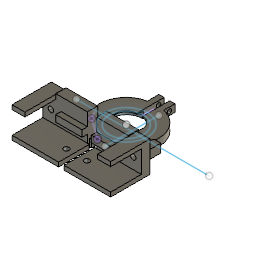
Tuisnlang to body koppelstuk (Autodesk Fusion 360 design; units mm, degrees)
part number: 2025-12-09-10-40-52-901
Autodesk Fusion 360 part; units mm, degrees
sketch "Sketch1" plane through (0, 0, 0) normal (0, 0, 1) x (1, 0, 0)
  circle A0 centre (0, 0) radius 25
  dimension "d1" = 50
  constraint coincident A0.centre origin
  measures "d1" diameter of A0
extrude "Extrude1" add sketch "Sketch1" along normal blind 2.6 makes body 1
sketch "Sketch2" plane through (0, 0, 2.6) normal (0, 0, 1) x (-1, 0, 0)
  circle A0 centre (0, 0) radius 25
  circle A1 centre (0, 0) radius 15
  dimension "d4" = 30
  constraint coincident A0.centre A1.centre
  measures "d4" diameter of A1
extrude "Extrude2" cut sketch "Sketch2" against normal blind 2.6 contours A1 bodies 1
sketch "Sketch3" plane through (0, 0, 0) normal (0, 1, 0) x (1, 0, 0)
sketch "Sketch5" plane through (0, 0, 0) normal (0, 0, 1) x (1, 0, 0)
  line L0 (-21.0001, -11.0728) -> (-21.84, -24.9305)
  line L1 (-21.84, -24.9305) -> (-16.242, -33.6943)
  line L2 (-16.242, -33.6943) -> (-1.8162, -24.4796)
  line L3 (-21.0001, -11.0728) -> (-1.8162, -24.4796)
  line L4 (-1.8162, -24.4796) -> (-1.8162, -34)
  line L5 (-1.8162, -34) -> (-31, -34)
  line L6 (-31, -34) -> (-31, -4.0843)
  line L7 (-31, -4.0843) -> (-25, -4.0843)
  line L8 (-25, -4.0843) -> (-21.0001, -11.0728)
  constraint perpendicular L1 L2
  constraint vertical L4
  constraint perpendicular L4 L5
  constraint perpendicular L5 L6
  constraint perpendicular L6 L7
extrude "Extrude3" add sketch "Sketch5" along normal blind 8 bodies 1
sketch "Sketch6" plane through (0, 0, 2.6) normal (0, 0, 1) x (-1, 0, 0)
  arc A0 (1.8162, 24.9339) -> (24.5053, 4.9486) centre (0, 0) ccw
  circle A1 centre (0, 0) radius 15
  circle A2 centre (32.676, 4.348) radius 1
  line L0 (24.5053, 4.9486) -> (21.0001, 11.0728)
  line L1 (21.0001, 11.0728) -> (1.8162, 24.4796)
  line L2 (1.8162, 24.4796) -> (1.8162, 24.9339)
  dimension "d9" = 2
  measures "d9" diameter of A2
extrude "Extrude4" cut sketch "Sketch6" against normal blind 2.6 contours A2 bodies 1
sketch "Sketch8" plane through (0, 0, 0) normal (0, 0, 1) x (1, 0, 0)
  line L0 (0, 25) -> (0, -25.7353)
  line L1 (0, -25.7353) -> (12.6085, -23.4951)
  line L2 (12.6085, -23.4951) -> (25, -10.7696)
  line L3 (25, -10.7696) -> (25, 9.1686)
  line L4 (25, 9.1686) -> (14.4225, 21.7368)
  line L5 (14.4225, 21.7368) -> (4.3268, 26.0635)
  line L6 (4.3268, 26.0635) -> (0, 25)
  constraint vertical L0
  constraint parallel L0 L3
extrude "Extrude5" cut sketch "Sketch8" along normal blind 19 bodies 1
sketch "Sketch9" plane through (0, 0, 0) normal (0, 0, 1) x (1, 0, 0)
  line L0 (4.9276, 25.1738) -> (4.9276, -24.4237)
  line L1 (-46, 0) -> (76.5197, 0)
  constraint vertical L0
  constraint horizontal L1
sketch "Sketch10" plane through (0, 0, 0) normal (0, 0, 1) x (1, 0, 0)
  spline S0 degree 5 poles (-0.4071, 24.1491) (-0.4918, 24.0205) (-0.6962, 23.8243) (-1.102, 23.7009) (-1.822, 23.7859) (-2.9658, 23.9832) (-4.2807, 23.9855) (-5.6641, 23.6781) (-7.0121, 23.0757) (-8.2499, 22.2797) (-9.3589, 21.4375) (-10.4145, 20.6984) (-11.5168, 20.2085) (-12.7525, 20.094) (-14.1577, 20.4469) (-15.6684, 21.3064) (-17.1289, 22.6564) (-18.3401, 24.4341) (-19.0952, 26.5352) (-19.2214, 28.8193) (-18.6168, 31.1155) (-17.296, 33.2264) (-15.3689, 34.9492) (-13.0093, 36.0992) (-10.4289, 36.5324) (-7.8486, 36.1699) (-5.4721, 35.0198) (-3.4561, 33.2063) (-1.8896, 30.981) (-0.8095, 28.6573) (-0.2122, 26.5558) (-0.0948, 25.268) (-0.1875, 24.5959) (-0.3223, 24.2778) (-0.4071, 24.1491) knots 0 0 0 0 0 0 0.033333 0.066667 0.1 0.133333 0.166667 0.2 0.233333 0.266667 0.3 0.333333 0.366667 0.4 0.433333 0.466667 0.5 0.533333 0.566667 0.6 0.633333 0.666667 0.7 0.733333 0.766667 0.8 0.833333 0.866667 0.9 0.933333 0.966667 1 1 1 1 1 1
  line L0 (-5.9786, 23.8802) -> (-11.3635, 20.0197)
  line L1 (-46, 0) -> (76.5197, 0)
  spline S1 degree 5 poles (-0.4071, -24.1491) (-0.4918, -24.0205) (-0.6962, -23.8243) (-1.102, -23.7009) (-1.822, -23.7859) (-2.9658, -23.9832) (-4.2807, -23.9855) (-5.6641, -23.6781) (-7.0121, -23.0757) (-8.2499, -22.2797) (-9.3589, -21.4375) (-10.4145, -20.6984) (-11.5168, -20.2085) (-12.7525, -20.094) (-14.1577, -20.4469) (-15.6684, -21.3064) (-17.1289, -22.6564) (-18.3401, -24.4341) (-19.0952, -26.5352) (-19.2214, -28.8193) (-18.6168, -31.1155) (-17.296, -33.2264) (-15.3689, -34.9492) (-13.0093, -36.0992) (-10.4289, -36.5324) (-7.8486, -36.1699) (-5.4721, -35.0198) (-3.4561, -33.2063) (-1.8896, -30.981) (-0.8095, -28.6573) (-0.2122, -26.5558) (-0.0948, -25.268) (-0.1875, -24.5959) (-0.3223, -24.2778) (-0.4071, -24.1491) knots 0 0 0 0 0 0 0.033333 0.066667 0.1 0.133333 0.166667 0.2 0.233333 0.266667 0.3 0.333333 0.366667 0.4 0.433333 0.466667 0.5 0.533333 0.566667 0.6 0.633333 0.666667 0.7 0.733333 0.766667 0.8 0.833333 0.866667 0.9 0.933333 0.966667 1 1 1 1 1 1
  line L2 (0.3754, 25.3361) -> (-1.1896, 22.9622)
  line L3 (0.3754, -25.3361) -> (-1.1896, -22.9622)
  line L4 (-5.9786, -23.8802) -> (-11.3635, -20.0197)
  point P0 (-3.0127, 23.9362)
  point P1 (-8.6711, 21.9499)
  point P2 (-13.3389, 20.2988)
  point P3 (-19, 29.1318)
  point P4 (-6, 35.1318)
  point P5 (-3.0127, -23.9362)
  point P6 (-8.6711, -21.9499)
  point P7 (-13.3389, -20.2988)
  point P8 (-19, -29.1318)
  point P9 (-6, -35.1318)
  constraint midpoint P1 L0
  constraint midpoint S0.start L2
  constraint symmetric S0.start L1 S1.start
  constraint symmetric P0 L1 P5
  constraint symmetric P1 L1 P6
  constraint symmetric P2 L1 P7
  constraint symmetric P3 L1 P8
  constraint symmetric P4 L1 P9
  constraint symmetric L0.start L1 L4.start
  constraint symmetric L0.end L1 L4.end
  constraint symmetric L1 L2.start L3.start
  constraint symmetric L1 L2.end L3.end
sketch "Sketch13" plane through (0, 0, 0) normal (0, 0, 1) x (1, 0, 0)
  line L0 (9.9066, 24.8111) -> (24.4111, 20.3394)
  line L1 (24.4111, 20.3394) -> (30.2441, 35.4836)
  line L2 (30.2441, 35.4836) -> (10.9741, 35.4836)
  line L3 (10.9741, 35.4836) -> (9.9066, 24.8111)
  line L4 (-46, 0) -> (76.5197, 0)
  line L5 (30.2441, -35.4836) -> (10.9741, -35.4836)
  line L6 (10.9741, -35.4836) -> (9.9066, -24.8111)
  line L7 (9.9066, -24.8111) -> (24.4111, -20.3394)
  line L8 (24.4111, -20.3394) -> (30.2441, -35.4836)
  constraint horizontal L2
  constraint symmetric L0.start L4 L6.end
  constraint symmetric L0.end L4 L7.end
  constraint symmetric L1.end L4 L5.start
  constraint symmetric L2.end L4 L5.end
sketch "Sketch19" plane through (0, 0, 2.6) normal (0, 0, 1) x (-1, 0, 0)
  line L0 (0, 25) -> (0, 15)
  arc A0 (0, -15) -> (0, 15) centre (0, 0) ccw
  arc A1 (0, -25) -> (24.5053, 4.9486) centre (0, 0) ccw
  circle A2 centre (0, 0) radius 15.7
  line L1 (0, -15) -> (0, -25)
  line L2 (24.5053, 4.9486) -> (21.0001, 11.0728)
  line L3 (21.0001, 11.0728) -> (1.8162, 24.4796)
  line L4 (1.8162, 24.4796) -> (1.8162, 24.9339)
  arc A3 (1.8162, 24.9339) -> (0, 25) centre (0, 0) ccw
  dimension "d25" = 31.4
  measures "d25" diameter of A2
sketch "Sketch20" plane through (0, 0, 2.6) normal (0, 0, 1) x (-1, 0, 0)
  line L0 (0, 25) -> (0, 15)
  arc A0 (0, -15) -> (0, 15) centre (0, 0) ccw
  arc A1 (0, -25) -> (24.5053, 4.9486) centre (0, 0) ccw
  circle A2 centre (0, 0) radius 19.4774
  circle A3 centre (0, 0) radius 15.7
  line L1 (0, -15) -> (0, -25)
  line L2 (24.5053, 4.9486) -> (21.0001, 11.0728)
  line L3 (21.0001, 11.0728) -> (1.8162, 24.4796)
  line L4 (1.8162, 24.4796) -> (1.8162, 24.9339)
  arc A4 (1.8162, 24.9339) -> (0, 25) centre (0, 0) ccw
  dimension "d30" = 31.4
  measures "d30" diameter of A3
extrude "Extrude12" add sketch "Sketch20" along normal blind 3.3 contours L0 A2 A3 L1 picked at (1.6688, 18.0989) bodies 1
sketch "Sketch21" plane through (0, 0, 5.9) normal (0, 0, 1) x (-1, 0, 0)
  arc A0 (0, -19.4774) -> (0, 19.4774) centre (0, 0) ccw
  line L0 (0, 19.4774) -> (0, 15.7)
  arc A1 (0, -15.7) -> (0, 15.7) centre (0, 0) ccw
  line L1 (0, -15.7) -> (0, -19.4774)
  circle A2 centre (0, 0) radius 19.4774
  constraint concentric A0 A2
extrude "Extrude13" add sketch "Sketch21" along normal blind 1 bodies 1
sketch "Sketch22" plane through (0, 0, 6.9) normal (0, 0, 1) x (-1, 0, 0)
  circle A0 centre (0, 0) radius 19.4774
  circle A1 centre (0, 0) radius 9.85
  dimension "d35" = 19.7
  constraint coincident A0.centre A1.centre
  measures "d35" diameter of A1
extrude "Extrude14" cut sketch "Sketch22" against normal blind 2 contours A1 bodies 1
extrude "Extrude15" add sketch "Sketch20" along normal blind 4.3 contours L0 A1 A2 L1 L2 L3 L4 A4 bodies 1
sketch "Sketch24" plane through (0, 0, 6.9) normal (0, 0, 1) x (-1, 0, 0)
  circle A0 centre (0, 0) radius 9.85
  arc A1 (0, 19.4774) -> (0, -19.4774) centre (0, 0) ccw
  line L0 (0, 24) -> (6, 24)
  line L1 (6, 24) -> (6, 32)
  line L2 (6, 32) -> (0, 32)
  line L3 (0, 32) -> (0, 24)
  line L4 (0, -19.4774) -> (0, -25)
  arc A2 (0, -25) -> (24.5053, 4.9486) centre (0, 0) ccw
  line L5 (0, 25) -> (0, 19.4774)
  line L6 (24.5053, 4.9486) -> (21.0001, 11.0728)
  line L7 (21.0001, 11.0728) -> (1.8162, 24.4796)
  line L8 (1.8162, 24.4796) -> (1.8162, 24.9339)
  arc A3 (1.8162, 24.9339) -> (0, 25) centre (0, 0) ccw
  constraint horizontal L0
  constraint vertical L1
  constraint horizontal L2
  constraint vertical L3
extrude "Extrude16" add sketch "Sketch24" against normal blind 6.9 contours L0 L3 L5 L7 L8 A3 | L0 L1 L2 L3 L7 L8 A3 bodies 1
sketch "Sketch25" plane through (0, 0, 0) normal (0, 0, 1) x (1, 0, 0)
  line L0 (0, 24.3391) -> (-5, 24.3391)
  line L1 (-5, 24.3391) -> (-5, 35.1439)
  line L2 (-5, 35.1439) -> (0, 35.1439)
  line L3 (0, 35.1439) -> (0, 24.3391)
  constraint horizontal L0
  constraint vertical L1
  constraint horizontal L2
  constraint vertical L3
extrude "Extrude17" add sketch "Sketch25" along normal blind 6.9 bodies 1
sketch "Sketch28" plane through (-31, 0, 0) normal (-1, 0, 0) x (0, -1, 0)
  line L0 (4.0843, 0) -> (34, 0)
  line L1 (34, 0) -> (34, 8)
  line L2 (34, 8) -> (4.0843, 8)
  line L3 (4.0843, 8) -> (4.0843, 0)
  line L4 (34, 8) -> (31, 8)
  line L5 (31, 8) -> (31, 0)
  line L6 (31, 0) -> (34, 0)
  line L7 (34, 0) -> (34, 8)
  constraint horizontal L4
  constraint vertical L5
  constraint horizontal L6
  constraint vertical L7
  constraint coincident L0 L5.end
  constraint coincident L1.end L2.start
extrude "Extrude19" add sketch "Sketch28" along normal blind 9 contours L0 L1 L2 L4 L5 L6 L7 bodies 1
sketch "Sketch29" plane through (0, -34, 0) normal (0, -1, 0) x (1, 0, 0)
  line L0 (-1.8162, 8) -> (-40, 8)
  line L1 (-40, 8) -> (-40, 0)
  line L2 (-40, 0) -> (-1.8162, 0)
  line L3 (-1.8162, 0) -> (-1.8162, 8)
  line L4 (-40, 4) -> (-31, 4)
  line L5 (-31, 4) -> (-31, 0)
  line L6 (-31, 0) -> (-40, 0)
  line L7 (-40, 0) -> (-40, 4)
  constraint horizontal L4
  constraint vertical L5
  constraint horizontal L6
  constraint vertical L7
  constraint coincident L2 L5.end
  constraint midpoint L1 L4.start
extrude "Extrude20" add sketch "Sketch29" along normal blind 12 contours L1 L2 L4 L5 L6 L7 bodies 1
sketch "Sketch30" plane through (0, 0, 8) normal (0, 0, 1) x (-1, 0, 0)
  line L0 (25, 4.0843) -> (31, 4.0843)
  line L1 (31, 4.0843) -> (31, 31)
  line L2 (31, 31) -> (40, 31)
  line L3 (40, 31) -> (40, 34)
  line L4 (40, 34) -> (1.8162, 34)
  line L5 (1.8162, 34) -> (1.8162, 24.4796)
  line L6 (1.8162, 24.4796) -> (21.0001, 11.0728)
  line L7 (21.0001, 11.0728) -> (25, 4.0843)
  line L8 (31, 31) -> (40, 31)
  line L9 (40, 31) -> (40, 34)
  line L10 (40, 34) -> (31, 34)
  line L11 (31, 34) -> (31, 31)
  constraint horizontal L8
  constraint vertical L9
  constraint horizontal L10
  constraint vertical L11
  constraint coincident L3.end L4.start
  constraint coincident L1.end L2.start
extrude "Extrude21" add sketch "Sketch30" along normal blind 16.4 contours L2 L3 L4 L8 L9 L10 L11 bodies 1
sketch "Sketch31" plane through (0, 0, 24.4) normal (0, 0, 1) x (-1, 0, 0)
  line L0 (31, 34) -> (31, 31)
  line L1 (31, 31) -> (40, 31)
  line L2 (40, 31) -> (40, 34)
  line L3 (40, 34) -> (31, 34)
  line L4 (31, 31) -> (40, 31)
  line L5 (40, 31) -> (40, 34)
  line L6 (40, 34) -> (31, 34)
  line L7 (31, 34) -> (31, 31)
  constraint horizontal L4
  constraint vertical L5
  constraint horizontal L6
  constraint vertical L7
  constraint coincident L2.end L3.start
  constraint coincident L0.end L1.start
extrude "Extrude22" add sketch "Sketch31" along normal blind 4 bodies 1
sketch "Sketch32" plane through (0, -34, 0) normal (0, -1, 0) x (1, 0, 0)
  line L0 (-40, 4) -> (-31, 4)
  line L1 (-1.8162, 0) -> (-1.8162, 8)
  line L2 (-1.8162, 8) -> (-31, 8)
  line L3 (-31, 8) -> (-31, 28.4)
  line L4 (-31, 28.4) -> (-40, 28.4)
  line L5 (-40, 28.4) -> (-40, 4)
  line L6 (-40, 28.4) -> (-31, 28.4)
  line L7 (-31, 28.4) -> (-31, 24.4)
  line L8 (-31, 24.4) -> (-40, 24.4)
  line L9 (-40, 24.4) -> (-40, 28.4)
  line L10 (-31, 4) -> (-31, 0)
  line L11 (-31, 0) -> (-1.8162, 0)
  dimension "d54" = 4
  constraint horizontal L6
  constraint vertical L7
  constraint horizontal L8
  constraint vertical L9
  constraint coincident L4.end L5.start
  measures "d54" distance of L4.end L8.end
extrude "Extrude23" add sketch "Sketch32" along normal blind 12 contours L3 L4 L5 L6 L7 L8 L9 bodies 1
sketch "Sketch34" plane through (0, 0, 6.9) normal (0, 0, 1) x (-1, 0, 0)
  arc A0 (5, -24.4949) -> (24.5053, 4.9486) centre (0, 0) ccw
  line L0 (24.5053, 4.9486) -> (21.0001, 11.0728)
  line L1 (21.0001, 11.0728) -> (1.8162, 24.4796)
  line L2 (1.8162, 24.4796) -> (1.8162, 32)
  line L3 (1.8162, 32) -> (0, 32)
  line L4 (0, 32) -> (0, 19.4774)
  arc A1 (0, 19.4774) -> (0, -19.4774) centre (0, 0) ccw
  line L5 (0, -19.4774) -> (0, -35.1439)
  line L6 (0, -35.1439) -> (5, -35.1439)
  line L7 (5, -35.1439) -> (5, -24.4949)
  circle A2 centre (0, 0) radius 9.85
  line L8 (0, 25) -> (-19.4774, 25)
  line L9 (-19.4774, 25) -> (-19.4774, -22.8796)
  line L10 (-19.4774, -22.8796) -> (0, -22.8796)
  line L11 (0, -22.8796) -> (0, 25)
  constraint horizontal L8
  constraint vertical L9
  constraint horizontal L10
  constraint vertical L11
  constraint coincident L4 L8.start
extrude "Extrude24" cut sketch "Sketch34" against normal blind 3 contours A1 L5 L9 L10 L11 | A1 A2 L11 | L4 A1 L8 L9 L11 | A2 L11 picked at (-2.567, 2.0471) bodies 1
sketch "Sketch35" plane through (0, 0, 8) normal (0, 0, 1) x (-1, 0, 0)
  line L0 (31, 31) -> (31, 34)
  line L1 (31, 34) -> (1.8162, 34)
  line L2 (1.8162, 34) -> (1.8162, 24.4796)
  line L3 (1.8162, 24.4796) -> (21.0001, 11.0728)
  line L4 (21.0001, 11.0728) -> (25, 4.0843)
  line L5 (25, 4.0843) -> (31, 4.0843)
  line L6 (31, 4.0843) -> (31, 31)
  line L7 (1.8162, 24.4796) -> (31, 24.4796)
  line L8 (31, 24.4796) -> (31, 34)
  line L9 (31, 34) -> (1.8162, 34)
  line L10 (1.8162, 34) -> (1.8162, 24.4796)
  constraint horizontal L7
  constraint vertical L8
  constraint horizontal L9
  constraint vertical L10
  constraint coincident L0.end L1.start
  constraint coincident L2.end L3.start
extrude "Extrude25" add sketch "Sketch35" along normal blind 21 contours L0 L1 L2 L6 L7 L8 L9 L10 bodies 1
sketch "Sketch36" plane through (0, -34, 0) normal (0, -1, 0) x (1, 0, 0)
  line L0 (-31, 24.4) -> (-40, 24.4)
  line L1 (-40, 24.4) -> (-40, 4)
  line L2 (-40, 4) -> (-31, 4)
  line L3 (-31, 4) -> (-31, 0)
  line L4 (-31, 0) -> (-1.8162, 0)
  line L5 (-1.8162, 0) -> (-1.8162, 29)
  line L6 (-1.8162, 29) -> (-31, 29)
  line L7 (-31, 29) -> (-31, 28.4)
  line L8 (-31, 28.4) -> (-31, 24.4)
  line L9 (-40, 14.2) -> (-1.8162, 14.2)
  line L10 (-26.0013, 17.2) -> (-26.0013, 10.4445)
  line L11 (-26.0013, 17.2) -> (-1.8162, 17.2)
  line L12 (-1.8162, 17.2) -> (-1.8162, 11.2)
  line L13 (-1.8162, 11.2) -> (-26.0013, 11.2)
  line L14 (-26.0013, 11.2) -> (-26.0013, 10.4445)
  line L15 (-1.8162, 10.4445) -> (-1.8162, 11.2)
  line L16 (-31, 24.4) -> (-1.8162, 24.4)
  line L17 (-1.8162, 24.4) -> (-1.8162, 17.2)
  line L18 (-31, 4) -> (-1.8162, 4)
  line L19 (-1.8162, 4) -> (-1.8162, 11.2)
  dimension "d61" = 6
  dimension "d62" = 7.2
  constraint midpoint L1 L9.start
  constraint coincident L5 L9.end
  constraint perpendicular L5 L9
  constraint perpendicular L9 L10
  constraint coincident L5 L11.end
  constraint perpendicular L5 L11
  constraint perpendicular L9 L12
  constraint horizontal L13
  constraint coincident L0.start L8.end
  constraint coincident L5 L16.end
  constraint perpendicular L5 L16
  constraint coincident L2.end L3.start
  constraint coincident L5 L18.end
  constraint perpendicular L5 L18
  measures "d61" distance of L11.end L12.end
  measures "d62" distance of L11.end L16.end
extrude "Extrude26" add sketch "Sketch36" along normal blind 5 contours L5 L9 L10 L11 L12 | L5 L9 L10 L12 L13 bodies 1
mirror "Mirror2" about plane through (0, 0, 0) normal (1, 0, 0) of bodies 1 makes body 2
move_body "Move3" bodies 2 to x (1, 0, 0) y (0, 1, 0) z (0, 0, 1) at (5, 0, 0)
hole "Hole1" at (10, 29.8194, 3.45) direction (-1, 0, 0) diameter 4 depth 20 tip angle 118 bodies 1 2
hole "Hole2" at (-35.5, -31, 14.2) direction (0, -1, 0) diameter 5 depth 6 tip angle 118 bodies 1
hole "Hole3" at (40.472, -31, 14.2) direction (0, -1, 0) diameter 5 depth 5 tip angle 118 bodies 2
extrude "Extrude27" add 2 faces at (-35.5, -31, 24.5) (40.4907, -31, 3.9) along direction (0, 1, 0) blind 5 on bodies 1 2 bodies 1 2
extrude "Extrude28" add 1 faces at (-40, -28.6667, 10.8) along direction (-1, 0, 0) blind 3 on bodies 1 bodies 1
extrude "Extrude29" add 1 faces at (45, -28.6667, 10.8) along direction (1, 0, 0) blind 3 on bodies 2 bodies 2
extrude "Extrude30" add 4 faces at (44, -46, 1.3333) (40, -46, 27.0667) (-35, -46, 27.0667) (-35, -46, 2.6667) along direction (0, -1, 0) blind 16.4 on bodies 1 2 bodies 2 1
extrude "Extrude31" add 1 faces at (-31, -43.4667, 2.6667) along direction (1, 0, 0) blind 31 on bodies 1 bodies 1
extrude "Extrude32" add 1 faces at (36, -43.4667, 2.6667) along direction (-1, 0, 0) blind 31 on bodies 2 bodies 2
hole "Hole6" at (42, -40.255, 0) direction (0, 0, 1) diameter 5 depth 6 tip angle 118 bodies 2
hole "Hole7" at (-37, -40.2, 0) direction (0, 0, 1) diameter 5 depth 6 tip angle 118 bodies 1
move_face "MoveFace1" to x (1, 0, 0) y (0, 1, 0) z (0, 0, 1) at (-30, -8, 0) 1 faces at (42.2489, -37.7674, 2.6667) on bodies 2
move_face "MoveFace2" to x (1, 0, 0) y (0, 1, 0) z (0, 0, 1) at (30, -8, 0) 1 faces at (-36.7511, -37.7124, 2.6667) on bodies 1
